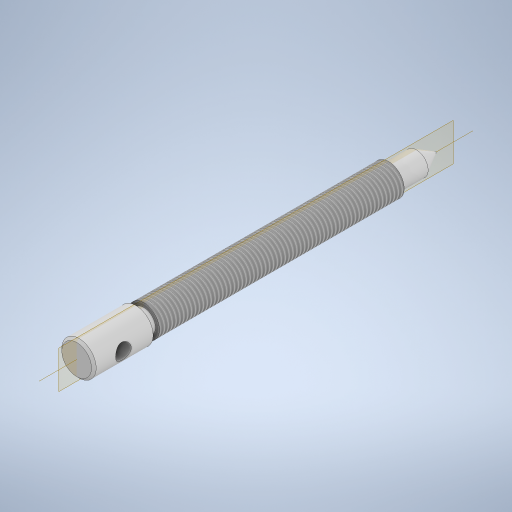
# Autodesk Inventor part: atividade_14A_eixo
Saved by Autodesk Inventor 2024.2 (Build 282272000, 272)
## iProperties
Created: 2024-03-04
Part Number: atividade_14A_eixo
Material: Generic
Document SubType Name: Modeling
Designer: 082220042
Density: 1 g/cm^3
Appearance: Default
Author: 082220042
Autodesk Inventor part; units mm, degrees
ref_plane "XZ Plane" through (0, 0, 0) normal (0, 1, 0) x (-1, 0, 0)
ref_plane "XY Plane" through (0, 0, 0) normal (0, 0, 1) x (1, 0, 0)
sketch "Sketch1" plane through (0, 0, 0) normal (1, 0, 0) x (0, 1, 0)
  line L0 (0, 0) -> (9.5, 0)
  line L1 (0, 0) -> (9.5, 0) construction
  line L2 (11, -1.5) -> (11, -38)
  line L3 (11, -38) -> (7.5, -38)
  line L4 (7.5, -38) -> (7.5, -43)
  line L5 (7.5, -43) -> (10, -43)
  line L6 (10, -43) -> (10, -200)
  line L7 (10, -200) -> (7.5, -200)
  line L8 (7.5, -200) -> (7.5, -217.8756)
  line L9 (0.5, -230) -> (0, -230)
  line L10 (0, -230) -> (0, 0)
  line L11 (0.5, -230) -> (7.5, -217.8756)
  line L12 (11, -1.5) -> (9.5, 0)
  line L13 (34.8708, -0.75) -> (56.3474, -0.75)
  line L14 (56.3474, -0.75) -> (56.3474, -28.5061)
  line L15 (56.3474, -28.5061) -> (34.8708, -28.5061)
  line L16 (34.8708, -28.5061) -> (34.8708, -0.75)
  point P0 (11, 0)
  point P1 (7.5, -230)
  point P2 (0.25, -230)
  dimension "d7" = 11
  dimension "d8" = 0
  dimension "d9" = 38
  dimension "d10" = 90
  dimension "d11" = 3.5
  dimension "d12" = 5
  dimension "d13" = 2.5
  dimension "d14" = 157
  dimension "d15" = 90
  dimension "d16" = 2.5
  dimension "d17" = 30
  dimension "d18" = 7.5
  dimension "d19" = 7.25
  dimension "d20" = 7
  dimension "d21" = 60
  dimension "d22" = 1.5
  dimension "d23" = 1.5
  constraints: 34 end point, 7 perpendicular, 6 point on line, 3 horizontal, 2 parallel, 1 collinear, 1 midpoint
  measures "d7" distance of L0.start point (11, 0)
  measures "d8" distance between parallel lines of L0 L1
  measures "d9" distance of point (11, 0) L2.end
  measures "d10" angle of L0 L2
  measures "d11" distance of L2.end L3.end
  measures "d12" distance of L3.end L4.end
  measures "d13" distance of L4.end L5.end
  measures "d14" distance of L5.end L6.end
  measures "d15" angle of L5 L6
  measures "d16" distance of L6.end L7.end
  measures "d17" distance of L7.end point (7.5, -230)
  measures "d18" distance of point (7.5, -230) L9.end
  measures "d19" distance from line of L8 point (0.25, -230)
  measures "d20" distance of L9.start point (7.5, -230)
  measures "d21" angle of L9 L11
  measures "d22" distance of L2.start point (11, 0)
  measures "d23" distance of L0.end point (11, 0)
revolve "Revolution1" add sketch "Sketch1" angle 360 about axis through (0, 0, -230) along (0, 0, 1) contours L0 L12 L2 L3 L4 L5 L6 L7 L8 L11 L9 L10
thread "Thread1" size "M20x2.5" class "6g" standard "ISO Metric profile" full length
sketch "Sketch4" plane through (0, 0, 0) normal (1, 0, 0) x (0, 1, 0)
  circle A0 centre (0, -19) radius 5
  line L0 (9.5, 0) -> (-9.5, 0) projected
  point P0 (0, 0)
  dimension "d27" = 10
  dimension "d28" = 19
  constraints: 1 centre point
  measures "d27" diameter of A0
  measures "d28" distance from line of L0 A0.centre
extrude "Extrusion1" cut sketch "Sketch4" along normal mid plane 40
equation "\"d23\" = d22"
body "Solid1"
